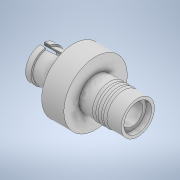
# Autodesk Inventor part: Axle
Saved by Autodesk Inventor 2020 (Build 240168000, 168)
## iProperties
Created: 2020-01-30
Part Number: Axle
Material: Generic
Document SubType Name: Modeling
Designer: cks4a449
Density: 1 g/cm^3
Appearance: Default
Author: cks4a449
Autodesk Inventor part; units mm, degrees
ref_plane "YZ Plane" through (0, 0, 0) normal (1, 0, 0) x (0, 1, 0)
ref_plane "XZ Plane" through (0, 0, 0) normal (0, 1, 0) x (-1, 0, 0)
ref_plane "XY Plane" through (0, 0, 0) normal (0, 0, 1) x (1, 0, 0)
sketch "Sketch1" plane through (0, 0, 0) normal (0, 0, 1) x (1, 0, 0)
  line L0 (22.6139, 7.6894) -> (22.6139, 6.2924)
  line L1 (0.7699, 6.2924) -> (0.7699, 7.6894)
  line L2 (11.9459, 3.8794) -> (12.9619, 3.8794)
  line L3 (12.9619, 3.8794) -> (12.9619, 6.2924)
  line L4 (11.9459, 6.2924) -> (11.9459, 3.8794)
  line L5 (11.9459, 6.2924) -> (0.7699, 6.2924)
  line L6 (12.1999, 7.6894) -> (12.1999, 9.7214)
  line L7 (12.1999, 11.1184) -> (12.9619, 11.1184)
  line L8 (12.9619, 11.1184) -> (12.9619, 7.6894)
  line L9 (12.9619, 11.1184) -> (7.8819, 11.1184)
  line L10 (7.8819, 11.1184) -> (7.8819, 9.7214)
  line L11 (7.8819, 9.7214) -> (12.1999, 9.7214)
  line L12 (12.9619, 9.7214) -> (12.9619, 11.1184)
  line L13 (11.9459, 3.8794) -> (0.9057, 3.8794)
  line L14 (0.7699, 7.6894) -> (2.0399, 7.6894)
  line L15 (2.0399, 7.6894) -> (2.0399, 7.3084)
  line L16 (0.7699, 7.6894) -> (2.0399, 7.6894)
  line L17 (7.1199, 7.6894) -> (2.0399, 7.3084)
  line L18 (0.7699, 7.6894) -> (2.0399, 7.6894)
  line L19 (7.1199, 7.6894) -> (12.1999, 7.6894)
  line L20 (18.1054, 7.8164) -> (17.4704, 7.8164)
  line L21 (17.4704, 6.1654) -> (18.1054, 7.8164) construction
  line L22 (18.1054, 6.1654) -> (17.4704, 7.8164) construction
  line L23 (16.8354, 7.8164) -> (16.2004, 7.8164)
  line L24 (16.2004, 6.1654) -> (16.8354, 7.8164) construction
  line L25 (16.8354, 6.1654) -> (16.2004, 7.8164) construction
  line L26 (19.3754, 7.8164) -> (18.7404, 7.8164)
  line L27 (18.7404, 6.1654) -> (19.3754, 7.8164) construction
  line L28 (19.3754, 6.1654) -> (18.7404, 7.8164) construction
  line L29 (16.2004, 7.8164) -> (16.2004, 7.6894)
  line L30 (16.8354, 7.6894) -> (16.8354, 7.8164)
  line L31 (17.4704, 7.8164) -> (17.4704, 7.6894)
  line L32 (18.1054, 7.6894) -> (18.1054, 7.8164)
  line L33 (18.7404, 7.8164) -> (18.7404, 7.6894)
  line L34 (19.3754, 7.6894) -> (19.3754, 7.8164)
  line L35 (19.3265, 7.6894) -> (22.6139, 7.6894)
  line L36 (22.6139, 6.2924) -> (19.3265, 6.2924)
  line L37 (18.0565, 7.6894) -> (18.7892, 7.6894)
  line L38 (12.9619, 7.6894) -> (16.2492, 7.6894)
  line L39 (16.7865, 7.6894) -> (17.5192, 7.6894)
  line L40 (19.3265, 6.2924) -> (16.2492, 6.2924)
  line L41 (16.7865, 6.2924) -> (12.9619, 6.2924)
  point P0 (16.2004, 6.2924)
  point P1 (16.8354, 6.2924)
  point P2 (17.4704, 6.2924)
  point P3 (19.3754, 6.2924)
  dimension "d8" = 21.844
  dimension "d9" = 1.397
  dimension "d10" = 11.176
  dimension "d12" = 11.43
  dimension "d13" = 12.192
  dimension "d15" = 12.192
  dimension "d16" = 7.239
  dimension "d17" = 1.397
  dimension "d18" = 7.112
  dimension "d34" = 1.27
  dimension "d35" = 0.381
  dimension "d36" = 6.35
  dimension "d38" = 0.635
  dimension "d39" = 1.651
  dimension "d41" = 0.635
  dimension "d42" = 1.651
  dimension "d44" = 0.635
  dimension "d45" = 1.651
  constraints: 84 end point, 32 parallel, 20 point on line, 9 horizontal, 9 perpendicular
  measures "d8" distance of L0.end L1.start
  measures "d9" distance of L0.start L0.end
  measures "d10" distance between parallel lines of L1 L4
  measures "d12" distance between parallel lines of L1 L6
  measures "d13" distance between parallel lines of L1 L8
  measures "d15" distance between parallel lines of L1 L3
  measures "d16" distance between parallel lines of L2 L7
  measures "d17" distance of L10.end L9.end
  measures "d18" distance between parallel lines of L1 L10
  measures "d34" distance of L14.end L1.end
  measures "d35" distance of L14.end L15.end
  measures "d36" distance of L1.end L17.start
  measures "d38" distance of L20.end L20.start
  measures "d39" distance of L20.start L22.start
  measures "d41" distance of L23.end L23.start
  measures "d42" distance of L23.start L25.start
  measures "d44" distance of L26.end L26.start
  measures "d45" distance of L26.start L28.start
revolve "Revolution1" add sketch "Sketch1" angle 360 about axis through (11.9459, 3.8794, 0) along (-1, 0, 0)
sketch "Sketch2" plane through (22.6139, 3.8794, 0) normal (1, 0, 0) x (0, 0, -1)
  circle A0 centre (0, 0) radius 3.175
  point P0 (0, -3.8794)
  dimension "d20" = 6.35
  constraints: 1 centre point
  measures "d20" diameter of A0
extrude "Extrusion1" cut sketch "Sketch2" against normal blind 1.27
sketch "Sketch3" plane through (0.7699, 3.8794, 0) normal (-1, 0, 0) x (0, 0, 1)
  circle A0 centre (0, 0) radius 3.175
  point P0 (0, -3.8794)
  dimension "d26" = 6.35
  constraints: 1 centre point
  measures "d26" diameter of A0
extrude "Extrusion2" cut sketch "Sketch3" against normal blind 6.35
sketch "Sketch4" plane through (0.7699, 3.8794, 0) normal (-1, 0, 0) x (0, 0, 1)
  line L0 (0.508, -9.525) -> (-0.508, -9.525)
  line L1 (-0.508, -9.525) -> (-0.508, 9.525)
  line L2 (-0.508, 9.525) -> (0.508, 9.525)
  line L3 (0.508, 9.525) -> (0.508, -9.525)
  line L4 (0.508, -9.525) -> (-0.508, 9.525) construction
  line L5 (-0.508, -9.525) -> (0.508, 9.525) construction
  point P0 (0, -3.8794)
  point P1 (0, 0)
  dimension "d30" = 1.016
  dimension "d31" = 19.05
  constraints: 12 end point, 2 midpoint, 2 parallel, 1 horizontal, 1 perpendicular
  measures "d30" distance of L1.end L2.end
  measures "d31" distance of L0.end L1.end
extrude "Extrusion3" cut sketch "Sketch4" against normal blind 5.08
chamfer "Chamfer1" distance 0.127 distance2 0.635 1 edges at (19.3754, -0.0576, 0) measured on face at (19.3754, 7.736, 0.3141)
chamfer "Chamfer2" distance 0.127 distance2 0.635 1 edges at (18.1054, -0.0576, 0) measured on face at (18.1054, 7.736, 0.3141)
chamfer "Chamfer3" distance 0.127 distance2 0.635 1 edges at (16.8354, -0.0576, 0) measured on face at (16.8354, 7.736, 0.3141)
body "Solid1"
